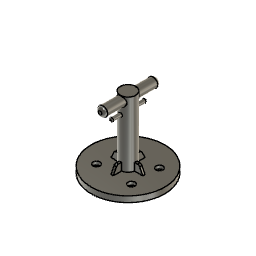
Robot Side v16 (Autodesk Fusion 360 design; units mm, degrees)
Autodesk Fusion 360 part; units mm, degrees
sketch "Sketch1" plane through (0, 0, 0) normal (0, 0, 1) x (1, 0, 0)
  line L0 (-25, 9) -> (-25, -9)
  line L1 (25, -9) -> (25, 9)
  line L2 (25, 9) -> (25, -9)
  line L3 (-25, -9) -> (-25, 9)
  ellipse E0 centre (-7.4315, -9) end of major axis (-25, -9) minor radius 15 (10.1172, -9.7125) -> (10.137, -9) ccw
  ellipse E1 centre (7.4315, -9) end of major axis (25, -9) minor radius 15 (7.4315, -24) -> (25, -9) ccw
  ellipse E2 centre (7.4315, -9) end of major axis (25, -9) minor radius 15 (-7.4315, -16.9977) -> (-5.8325, -18.8361) ccw
  ellipse E3 centre (7.4315, -9) end of major axis (25, -9) minor radius 15 (-10.137, -9) -> (-10.1172, -9.7125) ccw
  ellipse E4 centre (-7.4315, -9) end of major axis (-25, -9) minor radius 15 (-25, -9) -> (-7.4315, -24) ccw
  ellipse E5 centre (-7.4315, 9) end of major axis (-25, 9) minor radius 15 (-7.4315, 24) -> (-25, 9) ccw
  ellipse E6 centre (7.4315, 9) end of major axis (25, 9) minor radius 15 (25, 9) -> (7.4315, 24) ccw
  ellipse E7 centre (7.4315, 9) end of major axis (25, 9) minor radius 15 (-10.1172, 9.7125) -> (-10.137, 9) ccw
  circle A0 centre (14.9916, 12.0105) radius 3
  circle A1 centre (-14.9917, 12.0106) radius 3
  circle A2 centre (-14.9917, -12.0106) radius 3
  circle A3 centre (14.9916, -12.0105) radius 3
  line L4 (2.798, -22) -> (-2.798, -22)
  line L5 (-2.798, -22) -> (-2.798, -24)
  line L6 (2.798, -24) -> (2.798, -22)
  line L7 (-7.4315, -24) -> (-2.798, -24)
  line L8 (2.798, -24) -> (7.4315, -24)
  line L9 (-2.798, 22) -> (-2.798, 24)
  line L10 (2.798, 22) -> (-2.798, 22)
  line L11 (2.798, 24) -> (2.798, 22)
  line L12 (7.4315, 24) -> (2.798, 24)
  line L13 (-2.798, 24) -> (-7.4315, 24)
  circle A4 centre (14.9916, 12.0105) radius 1.6
  circle A5 centre (-14.9917, 12.0106) radius 1.6
  circle A6 centre (14.9916, -12.0105) radius 1.6
  circle A7 centre (-14.9917, -12.0106) radius 1.6
  circle A8 centre (0, 0) radius 31.5
  dimension "d3" = 50
  dimension "d4" = 18
  dimension "d5" = 14.863
  dimension "d6" = 48
  dimension "d12" = 6
  dimension "d14" = 6
  dimension "d19" = 3.2
  dimension "d20" = 3.2
  dimension "d59" = 63
  constraint parallel L0 L1
  constraint coincident A8.centre origin
  constraint parallel L2 L3
  constraint horizontal L12
  constraint parallel L7 L12
  constraint horizontal L4
  constraint perpendicular L4 L5
  constraint parallel L5 L6
  constraint collinear L7 L8
  constraint collinear L12 L13
  constraint concentric A0 A4
  constraint concentric A1 A5
  measures "d3" distance of L1.start L0.end
  measures "d4" distance of L1.end L1.start
  measures "d5" distance of L7.start L8.end
  measures "d6" distance of L13.end L7.start
  measures "d12" diameter of A0
  measures "d14" diameter of A1
  measures "d19" diameter of A4
  measures "d20" diameter of A5
  measures "d59" diameter of A8
extrude "Extrude1" add sketch "Sketch1" along normal blind 5 contours L0 L1 L2 L3 E1 E4 E5 E6 L4 L5 L6 L7 L8 L9 L10 L11 L12 L13 | A8 makes body 1
extrude "Extrude2" add sketch "Sketch1" along normal blind 2.19 contours A0 | A1 | A2 | A3 bodies 1
ref_plane "WorkPlane1" through (0, 0, 5) normal (0, 0, 1) x (1, 0, 0)
sketch "Sketch2" plane through (0, 0, 5) normal (0, 0, 1) x (1, 0, 0)
  circle A0 centre (0, 0) radius 6.65
  dimension "d24" = 13.3
  constraint coincident A0.centre origin
  measures "d24" diameter of A0
extrude "Extrude3" add sketch "Sketch2" along normal blind 58 bodies 1
ref_plane "WorkPlane2" through (0, -6.65, 36.3746) normal (0, -1, 0) x (-1, 0, 0)
sketch "Sketch3" plane through (0, -6.65, 0) normal (0, -1, 0) x (-1, 0, 0)
  circle A0 centre (0, -46.5) radius 1.65
  circle A1 centre (0, -56.5) radius 4.2
  line L0 (6.65, -60.7) -> (-6.65, -60.7)
  line L1 (-6.65, -63) -> (6.65, -63) construction
  line L2 (6.65, -5) -> (-6.65, -5) construction
  line L3 (-6.65, -63) -> (-6.65, -49.3707) construction
  line L4 (6.65, -63) -> (6.65, -55) construction
  line L5 (0, -60.7) -> (0, -63)
  dimension "d28" = 3.3
  dimension "d29" = 46.5
  dimension "d30" = 8.4
  dimension "d31" = 56.5
  constraint horizontal L0
  constraint tangent A1 L0
  constraint coincident L1.start L3.start
  constraint perpendicular L1 L3
  constraint coincident L0.end L3
  constraint coincident L1.end L4.start
  constraint perpendicular L1 L4
  constraint coincident L0.start L4
  constraint midpoint L0 L5.start
  constraint midpoint L1 L5.end
  constraint coincident A1.centre L5
  measures "d28" diameter of A0
  measures "d29" distance of origin A0.centre
  measures "d30" diameter of A1
  measures "d31" distance of origin A1.centre
extrude "Extrude6" cut sketch "Sketch3" against normal blind 21 bodies 1
extrude "Extrude9" cut 1 faces at (2.5195, 0.3798, 63) along direction (0, 0, -1) blind 2 on bodies 1 bodies 1
copy_body "Body->Comp2" bodies 1 removing the originals makes body 2 in component "Base"
sketch "Sketch1 (2)" plane through (0, 0, 0) normal (0, 1, 0) x (1, 0, 0) in component "Small Pin"
  circle A0 centre (35, 0) radius 1.5
  dimension "d40" = 3
  measures "d40" diameter of A0
extrude "Extrude1'" add sketch "Sketch1 (2)" along normal mid plane 30 separate body makes body 3 in component "Small Pin"
fillet "Fillet1" radius 1 2 edges at (33.6015, 15, 0.5424) (33.6015, -15, -0.5424) on bodies 3 in component "Small Pin"
sketch "Sketch1 (3)" plane through (0, 0, 0) normal (0, 1, 0) x (1, 0, 0) in component "Big Pin"
  circle A0 centre (-50, 0) radius 4
  dimension "d45" = 8
  measures "d45" diameter of A0
extrude "Extrude1''" add sketch "Sketch1 (3)" along normal mid plane 48 separate body makes body 4 in component "Big Pin"
fillet "Fillet1'" radius 2.5 2 edges at (-53.7293, 24, 1.4465) (-53.7293, -24, -1.4465) on bodies 4 in component "Big Pin"
sketch "Sketch5" plane through (0, 0, 0) normal (0, 1, 0) x (1, 0, 0)
  line L0 (6.65, -5) -> (-6.65, -5)
  spline S0 degree 3 poles (-4.2, -56.5) (-4.2, -55.9513) (-4.0871, -55.3837) (-3.6549, -54.3571) (-3.3357, -53.896) (-2.607, -53.1674) (-2.1451, -52.8461) (-1.1141, -52.412) (-0.5441, -52.3) (0.5441, -52.3) (1.1141, -52.412) (2.1451, -52.8461) (2.607, -53.1674) (3.3357, -53.896) (3.6549, -54.3571) (4.0871, -55.3837) (4.2, -55.9513) (4.2, -57.0487) (4.0871, -57.6163) (3.6549, -58.6429) (3.3357, -59.104) (2.607, -59.8326) (2.1451, -60.1539) (1.1141, -60.588) (0.5441, -60.7) (-0.5441, -60.7) (-1.1141, -60.588) (-2.1451, -60.1539) (-2.607, -59.8326) (-3.3357, -59.104) (-3.6549, -58.6429) (-4.0871, -57.6163) (-4.2, -57.0487) (-4.2, -56.5) knots 0 0 0 0 0.164599 0.164599 0.329199 0.329199 0.492427 0.492427 0.655655 0.655655 0.818884 0.818884 0.982112 0.982112 1.146711 1.146711 1.311311 1.311311 1.47591 1.47591 1.64051 1.64051 1.803738 1.803738 1.966966 1.966966 2.130195 2.130195 2.293423 2.293423 2.458022 2.458022 2.622622 2.622622 2.622622 2.622622
  spline S1 degree 3 poles (-1.65, -46.5) (-1.65, -46.2919) (-1.6082, -46.0705) (-1.4396, -45.6642) (-1.3127, -45.4793) (-1.0207, -45.1873) (-0.8358, -45.0604) (-0.4295, -44.8918) (-0.2081, -44.85) (0.2081, -44.85) (0.4295, -44.8918) (0.8358, -45.0604) (1.0207, -45.1873) (1.3127, -45.4793) (1.4396, -45.6642) (1.6082, -46.0705) (1.65, -46.2919) (1.65, -46.7081) (1.6082, -46.9295) (1.4396, -47.3358) (1.3127, -47.5207) (1.0207, -47.8127) (0.8358, -47.9396) (0.4295, -48.1082) (0.2081, -48.15) (-0.2081, -48.15) (-0.4295, -48.1082) (-0.8358, -47.9396) (-1.0207, -47.8127) (-1.3127, -47.5207) (-1.4396, -47.3358) (-1.6082, -46.9295) (-1.65, -46.7081) (-1.65, -46.5) knots 0 0 0 0 0.062439 0.062439 0.124879 0.124879 0.18731 0.18731 0.249741 0.249741 0.312172 0.312172 0.374603 0.374603 0.437042 0.437042 0.499481 0.499481 0.561921 0.561921 0.62436 0.62436 0.686791 0.686791 0.749222 0.749222 0.811653 0.811653 0.874084 0.874084 0.936523 0.936523 0.998963 0.998963 0.998963 0.998963
  line L1 (6.65, -5) -> (6.65, -11.5)
  line L2 (6.65, -11.5) -> (9.1678, -11.5)
  line L3 (10.9566, -10.3944) -> (13.6538, -5)
  line L4 (13.6538, -5) -> (6.65, -5)
  arc A0 (9.1678, -11.5) -> (10.9566, -10.3944) centre (9.1678, -9.5) ccw
  spline S2 degree 3 poles (0, -60.7) (0.5441, -60.7) (1.1141, -60.588) (2.1451, -60.1539) (2.607, -59.8326) (3.3357, -59.104) (3.6549, -58.6429) (4.0871, -57.6163) (4.2, -57.0487) (4.2, -55.9513) (4.0871, -55.3837) (3.6549, -54.3571) (3.3357, -53.896) (2.607, -53.1674) (2.1451, -52.8461) (1.1141, -52.412) (0.5441, -52.3) (0, -52.3) knots 0.655655 0.655655 0.655655 0.655655 0.818884 0.818884 0.982112 0.982112 1.146711 1.146711 1.311311 1.311311 1.47591 1.47591 1.64051 1.64051 1.803738 1.803738 1.966966 1.966966 1.966966 1.966966
  spline S3 degree 3 poles (0, -48.15) (0.2081, -48.15) (0.4295, -48.1082) (0.8358, -47.9396) (1.0207, -47.8127) (1.3127, -47.5207) (1.4396, -47.3358) (1.6082, -46.9295) (1.65, -46.7081) (1.65, -46.2919) (1.6082, -46.0705) (1.4396, -45.6642) (1.3127, -45.4793) (1.0207, -45.1873) (0.8358, -45.0604) (0.4295, -44.8918) (0.2081, -44.85) (0, -44.85) knots 0.249741 0.249741 0.249741 0.249741 0.312172 0.312172 0.374603 0.374603 0.437042 0.437042 0.499481 0.499481 0.561921 0.561921 0.62436 0.62436 0.686791 0.686791 0.749222 0.749222 0.749222 0.749222
  line L5 (6.65, -61) -> (-6.65, -61)
  spline S4 degree 3 poles (0, -44.85) (-0.2081, -44.85) (-0.4295, -44.8918) (-0.8358, -45.0604) (-1.0207, -45.1873) (-1.3127, -45.4793) (-1.4396, -45.6642) (-1.6082, -46.0705) (-1.65, -46.2919) (-1.65, -46.5) (-1.65, -46.7081) (-1.6082, -46.9295) (-1.4396, -47.3358) (-1.3127, -47.5207) (-1.0207, -47.8127) (-0.8358, -47.9396) (-0.4295, -48.1082) (-0.2081, -48.15) (0, -48.15) knots 0.749222 0.749222 0.749222 0.749222 0.811653 0.811653 0.874084 0.874084 0.936523 0.936523 0.998963 0.998963 0.998963 1.061402 1.061402 1.123842 1.123842 1.186272 1.186272 1.248703 1.248703 1.248703 1.248703
  spline S5 degree 3 poles (0, -52.3) (-0.5441, -52.3) (-1.1141, -52.412) (-2.1451, -52.8461) (-2.607, -53.1674) (-3.3357, -53.896) (-3.6549, -54.3571) (-4.0871, -55.3837) (-4.2, -55.9513) (-4.2, -56.5) (-4.2, -57.0487) (-4.0871, -57.6163) (-3.6549, -58.6429) (-3.3357, -59.104) (-2.607, -59.8326) (-2.1451, -60.1539) (-1.1141, -60.588) (-0.5441, -60.7) (0, -60.7) knots 1.966966 1.966966 1.966966 1.966966 2.130195 2.130195 2.293423 2.293423 2.458022 2.458022 2.622622 2.622622 2.622622 2.787221 2.787221 2.951821 2.951821 3.115049 3.115049 3.278277 3.278277 3.278277 3.278277
  dimension "d65" = 2
  dimension "d72" = 6.5
  dimension "d73" = 7.0038
  constraint coincident L0.start L1.start
  constraint perpendicular L0 L1
  constraint perpendicular L1 L2
  constraint tangent L2 A0
  constraint tangent L3 A0
  constraint parallel L2 L4
  measures "d65" radius of A0
  measures "d72" distance of L0.start L1.end
  measures "d73" distance of L0.start L3.end
extrude "Extrude7" add sketch "Sketch5" along normal mid plane 2 separate body contours L1 L2 L3 L4 A0 makes body 5
extrude "Extrude8" add 1 faces at (6.65, 0.3333, 9.3333) along direction (-1, 0, 0) blind 0.3 on bodies 5 bodies 5
pattern_circular "C-Pattern1" count 4 over 360 about axis through (0, 0, -23.25) along (0, 0, 1) of bodies 5 makes body 6 at (-1, 10.4202, 6.7981) makes body 7 at (-10.4202, -1, 6.7981) makes body 8 at (1, -10.4202, 6.7981)
combine "Combine1" operation add target body 2 tool bodies 5 6 7 8 in component "Base"
extrude "Extrude2'" cut 1 faces at (2.5195, 0.3798, 61) along direction (0, 0, -1) blind 0.1 on bodies 2 bodies 2 in component "Base"
component "Small Pin" placed x (1, 0, 0) y (0, 1, 0) z (0, 0, 1) at (-35, 0, 46.5)
component "Big Pin" placed x (1, 0, 0) y (0, 1, 0) z (0, 0, 1) at (50, 0, 56.5)
component "Base" placed x (1, 0, 0) y (0, 1, 0) z (0, 0, 1) at (0, 0, 0)
equation "d21 = 5 mm - 2.81 mm"
equation "d24 = ( 13.3 * Ratio ) * 1 mm"
equation "d41 = ( 30 * Ratio ) * 1 mm"
equation "d46 = ( 48 * Ratio ) * 1 mm"
equation "Ratio = 63 / 63"
